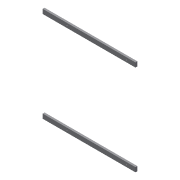
# Autodesk Inventor part: Node_location_jig
Saved by Autodesk Inventor 2017 (Build 210142000, 142)
## iProperties
Created: 2018-04-20
Part Number: Node_location_jig
Material: Generic
Document SubType Name: Modeling
Designer: Kathryn Rosie
Density: 1 g/cm^3
Appearance: Default
Author: Kathryn Rosie
Autodesk Inventor part; units mm, degrees
ref_plane "YZ Plane" through (0, 0, 0) normal (1, 0, 0) x (0, 1, 0)
ref_plane "XZ Plane" through (0, 0, 0) normal (0, 1, 0) x (-1, 0, 0)
ref_plane "XY Plane" through (0, 0, 0) normal (0, 0, 1) x (1, 0, 0)
sketch "Sketch1" plane through (0, 0, 0) normal (0, 0, 1) x (1, 0, 0)
  line L0 (22, 0) -> (22, -1544) projected
  circle A0 centre (-290, -632) radius 55 projected
  line L1 (-1022, -1544) -> (-1022, 0) projected
  line L2 (22, -147) -> (-1022, -147)
  line L3 (-1022, -147) -> (-1022, -97)
  line L4 (-1022, -97) -> (22, -97)
  line L5 (22, -97) -> (22, -147)
  line L6 (-290, -632) -> (22, -632) construction
  line L7 (-1022, -122) -> (22, -122) construction
  circle A1 centre (-80, -122) radius 6
  circle A2 centre (-750, -122) radius 6
  line L8 (22, -1117) -> (-1022, -1117)
  line L9 (-1022, -1117) -> (-1022, -1167)
  line L10 (-1022, -1167) -> (22, -1167)
  line L11 (22, -1167) -> (22, -1117)
  line L12 (-1022, -1142) -> (22, -1142) construction
  circle A3 centre (-80, -1142) radius 6
  circle A4 centre (-750, -1142) radius 6
  point P0 (0, 0)
  dimension "d0" = 50
  dimension "d1" = 510
  dimension "d2" = 12
  dimension "d3" = 210
  dimension "d7" = 12
  dimension "d8" = 670
  constraints: 22 end point, 8 symmetric about line, 7 point on line, 4 centre point, 2 midpoint, 2 parallel, 2 perpendicular, 1 horizontal, 2 other
  measures "d0" distance between parallel lines of L4 L2
  measures "d1" distance from line of L7 L6.start
  measures "d2" diameter of A1
  measures "d3" horizontal distance of L6.start A1.centre
  measures "d7" diameter of A2
  measures "d8" distance of A1.centre A2.centre
extrude "Extrusion1" add sketch "Sketch1" along normal blind 22 contours L0 L2 L1 L4 | L0 L10 L1 L8
body "Solid1"
